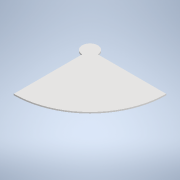
# Autodesk Inventor part: ramp
Saved by Autodesk Inventor 2021 (Build 250183000, 183)
## iProperties
Created: 2020-09-12
Part Number: ramp
Material: Generic
Document SubType Name: Modeling
Designer: deli
Density: 1 g/cm^3
Appearance: Default
Author: deli
Autodesk Inventor part; units mm, degrees
ref_plane "YZ Plane" through (0, 0, 0) normal (1, 0, 0) x (0, 1, 0)
ref_plane "XZ Plane" through (0, 0, 0) normal (0, 1, 0) x (-1, 0, 0)
ref_plane "XY Plane" through (0, 0, 0) normal (0, 0, 1) x (1, 0, 0)
sketch "Sketch1" plane through (0, 0, 0) normal (0, 1, 0) x (-1, 0, 0)
  arc A0 (40.8631, 289.0847) -> (-143.2869, 104.9347) centre (40.8631, 104.9347) ccw
  line L0 (21.8131, 104.9347) -> (-143.2869, 104.9347)
  line L1 (40.8631, 289.0847) -> (40.8631, 123.9847)
  arc A1 (21.8131, 104.9347) -> (40.8631, 123.9847) centre (40.8631, 104.9347) ccw
  point P0 (0, 0)
  dimension "d0" = 368.3
  dimension "d2" = 0
  dimension "d3" = 38.1
  constraints: 4 end point, 4 point on circle, 2 centre point, 1 horizontal, 1 vertical
  measures "d0" diameter of A0
  measures "d2" distance from line of A0.centre L0
  measures "d3" diameter of A1
extrude "Extrusion1" add sketch "Sketch1" along normal blind 3.175
body "Solid1"
